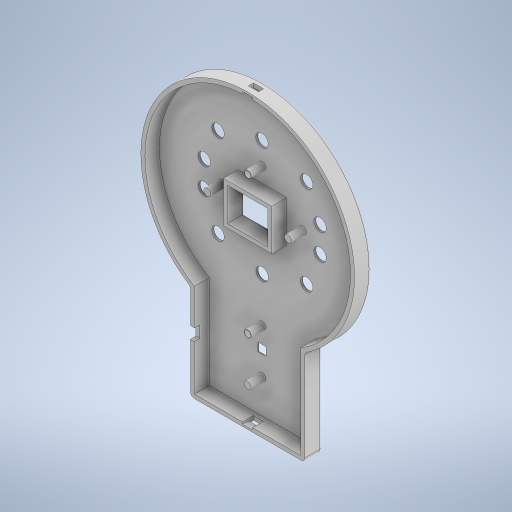
# Autodesk Inventor part: TopBox
Saved by Autodesk Inventor 2024 (Build 280153000, 153)
## iProperties
Created: 2023-11-16
Part Number: TopBox
Material: Générique
Document SubType Name: Modeling
Designer: digiacom
Density: 1 g/cm^3
Appearance: Par défaut
Author: digiacom
Autodesk Inventor part; units mm, degrees
ref_plane "YZ Plane" through (0, 0, 0) normal (1, 0, 0) x (0, 1, 0)
ref_plane "XZ Plane" through (0, 0, 0) normal (0, 1, 0) x (-1, 0, 0)
ref_plane "XY Plane" through (0, 0, 0) normal (0, 0, 1) x (1, 0, 0)
sketch "Esquisse1" plane through (0, 0, 0) normal (0, 0, 1) x (1, 0, 0)
  circle A0 centre (0, 0) radius 51
  line L0 (0, 0) -> (-26.4, 0)
  line L1 (-26.4, 0) -> (-26.4, -90)
  line L2 (-26.4, -90) -> (0, -90)
  line L3 (0, -90) -> (0, 0)
  line L4 (0, 0) -> (26.4, 0)
  line L5 (26.4, 0) -> (26.4, -90)
  line L6 (26.4, -90) -> (0, -90)
  line L7 (0, -90) -> (0, 0)
  point P0 (26.4, -43.6353)
  point P1 (-26.4, -43.6353)
  dimension "d5" = 102
  dimension "d6" = 26.4
  dimension "d7" = 90
  dimension "d8" = 26.4
  constraints: 16 end point, 4 parallel, 2 horizontal, 2 perpendicular, 1 centre point, 1 coincident, 1 point on line
  measures "d5" diameter of A0
  measures "d6" distance of L2.end L1.end
  measures "d7" distance of L1.end L0.end
  measures "d8" distance of L5.end L6.end
extrude "Extrusion2" add sketch "Esquisse1" along normal blind 1
sketch "Esquisse2" plane through (0, 0, 1) normal (0, 0, 1) x (1, 0, 0)
  circle A0 centre (0, -50.9) radius 1.75
  line L0 (-26.4, -90) -> (26.4, -90) projected
  line L1 (-26.4, -43.6353) -> (-26.4, -90) projected
  circle A1 centre (0, 17.68) radius 1.75
  point P0 (0, 0)
  dimension "d11" = 3.5
  dimension "d12" = 39.1
  dimension "d13" = 26.4
  dimension "d19" = 3.5
  dimension "d20" = 107.68
  dimension "d21" = 26.4
  constraints: 2 centre point
  measures "d11" diameter of A0
  measures "d12" distance from line of L0 A0.centre
  measures "d13" distance from line of L1 A0.centre
  measures "d19" diameter of A1
  measures "d20" distance from line of L0 A1.centre
  measures "d21" distance from line of L1 A1.centre
extrude "Extrusion5" add sketch "Esquisse2" along normal blind 7.195
sketch "Esquisse4" plane through (0, -50.9, 8.195) normal (0, 0, 1) x (1, 0, 0)
  circle A0 centre (0, 0) radius 1.5
  point P0 (0, 50.9)
  dimension "d24" = 3
  constraints: 1 centre point
  measures "d24" diameter of A0
sketch "Esquisse5" plane through (0, 17.68, 8.195) normal (0, 0, 1) x (1, 0, 0)
  circle A0 centre (0, 0) radius 1.75 projected
  circle A1 centre (0, 0) radius 1.5
  point P0 (0, -17.68)
  dimension "d25" = 3
  constraints: 1 centre point, 1 coincident
  measures "d25" diameter of A1
extrude "Extrusion6" cut sketch "Esquisse4" against normal blind 3
extrude "Extrusion7" cut sketch "Esquisse5" against normal blind 3 contours A1
sketch "Esquisse6" plane through (0, 0, 1) normal (0, 0, 1) x (1, 0, 0)
  circle A0 centre (0, -73) radius 1.75
  line L0 (-26.4, -90) -> (26.4, -90) projected
  circle A1 centre (20, 0) radius 1.75
  circle A2 centre (-20, 0) radius 1.75
  point P0 (0, 0)
  dimension "d30" = 3.5
  dimension "d31" = 17
  dimension "d32" = 3.5
  dimension "d33" = 3.5
  dimension "d34" = 20
  dimension "d37" = 20
  constraints: 3 centre point
  measures "d30" diameter of A0
  measures "d31" distance from line of L0 A0.centre
  measures "d32" diameter of A1
  measures "d33" diameter of A2
  measures "d34" distance of point (0, 0) A1.centre
  measures "d37" distance of point (0, 0) A2.centre
extrude "Extrusion8" add sketch "Esquisse6" along normal blind 7.195
sketch "Esquisse8" plane through (0, 0, 0) normal (0, 0, -1) x (-1, 0, 0)
  circle A0 centre (0, 0) radius 53
  circle A1 centre (0, 0) radius 51
  line L0 (-26.4, -90) -> (-26.4, -43.6353) projected
  line L1 (-26.4, -90) -> (26.4, -90)
  line L2 (26.4, -90) -> (26.4, -35.4414)
  line L3 (26.4, -35.4414) -> (-26.4, -35.4414)
  line L4 (-26.4, -35.4414) -> (-26.4, -90)
  line L5 (-28.4, -92) -> (28.4, -92)
  line L6 (28.4, -92) -> (28.4, -28.7229)
  line L7 (28.4, -28.7229) -> (-28.4, -28.7229)
  line L8 (-28.4, -28.7229) -> (-28.4, -92)
  point P0 (26.4, -43.6353)
  point P1 (28.4, -44.7486)
  point P2 (-28.4, -44.7486)
  dimension "d39" = 102
  dimension "d38" = 106
  dimension "d40" = 2
  dimension "d41" = 2
  dimension "d42" = 2
  constraints: 16 end point, 4 parallel, 2 coincident, 2 horizontal, 2 perpendicular, 1 centre point, 2 other
  measures "d38" diameter of A0
  measures "d40" distance between parallel lines of L8 L0
  measures "d41" distance between parallel lines of L5 L1
  measures "d42" distance between parallel lines of L2 L6
extrude "Extrusion9" add sketch "Esquisse8" against normal blind 8.195 contours A0 L6 A1 L8 | L8 A1 L0 A0 | A0 L0 L1 L2 L6 L5 L8 | A0 L2 A1 L6
fillet "Congé1" radius 1 4 edges at (0, 53, 0) (28.4, -68.3743, 0) (0, -92, 0) (-28.4, -68.3743, 0)
fillet "Congé2" radius 2 8 edges at (28.0904, -44.5781, 0.2766) (28.4, -44.7486, 4.5975) (28.1071, -91.7071, 0.2929) (28.4, -92, 4.5975) (-28.1071, -91.7071, 0.2929) (-28.4, -92, 4.5975) (-28.0904, -44.5781, 0.2766) (-28.4, -44.7486, 4.5975)
sketch "Esquisse9" plane through (0, 0, 1) normal (0, 0, 1) x (1, 0, 0)
  circle A0 centre (0, -28.8) radius 3.05
  line L0 (26.4, -90) -> (-26.4, -90) projected
  circle A1 centre (22.085, -22.12) radius 3.05
  arc A2 (26.4, -43.6353) -> (-26.4, -43.6353) centre (0, 0) ccw projected
  line L1 (-50.095, 49.99) -> (50.095, 49.99)
  line L2 (50.095, 49.99) -> (50.095, -89)
  line L3 (50.095, -89) -> (-50.095, -89)
  line L4 (-50.095, -89) -> (-50.095, 49.99)
  arc A3 (29.2945, -44.1682) -> (-29.2945, -44.1682) centre (0, 0) ccw projected
  circle A4 centre (28.705, -6) radius 3.05
  circle A5 centre (28.705, 6.75) radius 3.05
  circle A6 centre (22.085, 22) radius 3.05
  circle A7 centre (-0.1, 28.6) radius 3.05
  circle A8 centre (-21.915, 21.89) radius 3.05
  circle A9 centre (-28.705, 6.25) radius 3.05
  circle A10 centre (-28.705, -6.5) radius 3.05
  circle A11 centre (-21.915, -22.32) radius 3.05
  point P0 (50.095, -19.505)
  dimension "d47" = 6.1
  dimension "d48" = 0
  dimension "d49" = 61.2
  dimension "d52" = 6.1
  dimension "d55" = 50.095
  dimension "d56" = 50.095
  dimension "d57" = 28.01
  dimension "d58" = 138.99
  dimension "d59" = 1
  dimension "d60" = -49.99
  dimension "d61" = 66.88
  dimension "d62" = 6.1
  dimension "d63" = 21.39
  dimension "d64" = 83
  dimension "d65" = 6.1
  dimension "d66" = 95.75
  dimension "d67" = 6.1
  dimension "d68" = 111
  dimension "d69" = 6.1
  dimension "d70" = 117.6
  dimension "d71" = 50.195
  dimension "d72" = 6.1
  dimension "d73" = 28.18
  dimension "d74" = 28.1
  dimension "d75" = 6.1
  dimension "d76" = 21.39
  dimension "d77" = 95.25
  dimension "d78" = 6.1
  dimension "d79" = 83.5
  dimension "d80" = 6.1
  dimension "d81" = 66.68
  constraints: 10 centre point, 8 end point, 2 parallel, 1 horizontal, 1 midpoint, 1 perpendicular
  measures "d47" diameter of A0
  measures "d48" horizontal distance of point (0, 0) A0.centre
  measures "d49" distance from line of L0 A0.centre
  measures "d52" diameter of A1
  measures "d55" horizontal distance of point (50.095, -19.505) A3.centre
  measures "d56" distance from line of point (0, 0) L4
  measures "d57" distance from line of L2 A1.centre
  measures "d58" distance between parallel lines of L3 L1
  measures "d59" distance between parallel lines of L0 L3
  measures "d60" distance from line of A2.centre L1
  measures "d61" distance from line of L3 A1.centre
  measures "d62" diameter of A4
  measures "d63" distance from line of L2 A4.centre
  measures "d64" distance from line of L3 A4.centre
  measures "d65" diameter of A5
  measures "d66" distance from line of L3 A5.centre
  measures "d67" diameter of A6
  measures "d68" distance from line of L3 A6.centre
  measures "d69" diameter of A7
  measures "d70" distance from line of L3 A7.centre
  measures "d71" distance from line of A7.centre L2
  measures "d72" diameter of A8
  measures "d73" distance from line of L4 A8.centre
  measures "d74" distance from line of A8.centre L1
  measures "d75" diameter of A9
  measures "d76" distance from line of L4 A9.centre
  measures "d77" distance from line of A9.centre L3
  measures "d78" diameter of A10
  measures "d79" distance from line of L0 A10.centre
  measures "d80" diameter of A11
  measures "d81" distance from line of L3 A11.centre
extrude "Extrusion10" cut sketch "Esquisse9" against normal blind 2 contours A0 | A1 | A4 | A5 | A6 | A7 | A8 | A9 | A10 | A11
sketch "Esquisse10" plane through (-28.4, -90, 1) normal (-1, 0, 0) x (0, 0, 1)
  point P0 (-1, 90)
sketch "Esquisse11" plane through (-28.4, -90, 1) normal (-1, 0, 0) x (0, 0, 1)
  line L0 (7.195, 46.3647) -> (7.195, 0) projected
  line L1 (7.195, 22.55) -> (4.495, 22.55)
  line L2 (4.495, 22.55) -> (4.495, 28.45)
  line L3 (4.495, 28.45) -> (7.195, 28.45)
  line L4 (7.195, 28.45) -> (7.195, 22.55)
  line L5 (7.195, 0) -> (0, 0) projected
  point P0 (-1, 90)
  point P1 (5.845, 28.45)
  point P2 (7.195, 28.45)
  dimension "d82" = 28.45
  dimension "d83" = 5.9
  dimension "d84" = 2.7
  constraints: 8 end point, 2 parallel, 1 horizontal, 1 midpoint, 1 perpendicular, 1 point on line
  measures "d82" distance between parallel lines of L3 L5
  measures "d83" distance from line of point (5.845, 28.45) L1
  measures "d84" distance between parallel lines of L0 L2
extrude "Extrusion11" cut sketch "Esquisse11" against normal blind 2
sketch "Esquisse12" plane through (0, 0, 0) normal (0, 0, -1) x (-1, 0, 0)
  line L0 (-1.9, -59.1) -> (2.1, -59.1)
  line L1 (2.1, -59.1) -> (2.1, -63.1)
  line L2 (2.1, -63.1) -> (-1.9, -63.1)
  line L3 (-1.9, -63.1) -> (-1.9, -59.1)
  line L4 (-28.4, -45.8349) -> (-28.4, -90) projected
  line L5 (-26.4, -92) -> (26.4, -92) projected
  point P0 (0, 0)
  point P1 (2.1, -61.1)
  point P2 (-1.9, -61.1)
  point P3 (0.1, -63.1)
  point P4 (0.1, -59.1)
  dimension "d87" = 4
  dimension "d88" = 26.5
  dimension "d89" = 4
  dimension "d90" = 28.9
  constraints: 8 end point, 4 midpoint, 2 parallel, 1 horizontal, 1 perpendicular
  measures "d87" distance from line of point (2.1, -61.1) L3
  measures "d88" distance from line of L4 point (-1.9, -61.1)
  measures "d89" distance of point (0.1, -63.1) point (0.1, -59.1)
  measures "d90" distance between parallel lines of L5 L2
extrude "Extrusion12" cut sketch "Esquisse12" against normal blind 1
fillet "Congé3" radius 1 4 edges at (1.9, -61.1, 0) (-0.1, -59.1, 0) (-0.1, -63.1, 0) (-2.1, -61.1, 0)
sketch "Esquisse13" plane through (-26.4, -92, 1) normal (0, -1, 0) x (1, 0, 0)
  line L0 (23.9, 4.317) -> (28.9, 4.317)
  line L1 (28.9, 4.317) -> (28.9, 1.817)
  line L2 (28.9, 1.817) -> (23.9, 1.817)
  line L3 (23.9, 1.817) -> (23.9, 4.317)
  line L4 (-2.8945, 7.195) -> (-2.8945, 0) projected
  line L5 (55.6945, 0) -> (55.6945, 7.195) projected
  line L6 (0, 7.195) -> (52.8, 7.195) projected
  point P0 (26.4, -1)
  point P1 (-2.8945, 3.5975)
  point P2 (23.9, 3.067)
  point P3 (55.6945, 3.5975)
  point P4 (26.4, 1.817)
  point P5 (26.4, 4.317)
  dimension "d94" = 26.7945
  dimension "d95" = 5
  dimension "d96" = 26.7946
  dimension "d97" = 2.5
  dimension "d98" = 2.878
  constraints: 8 end point, 5 midpoint, 2 parallel, 1 horizontal, 1 perpendicular
  measures "d94" horizontal distance of point (-2.895, 3.598) point (23.9, 3.067)
  measures "d95" distance between parallel lines of L1 L3
  measures "d96" distance from line of point (55.695, 3.598) L1
  measures "d97" distance of point (26.4, 1.817) point (26.4, 4.317)
  measures "d98" distance between parallel lines of L6 L0
extrude "Extrusion13" cut sketch "Esquisse13" against normal blind 2
sketch "Esquisse14" plane through (0, 0, 8.195) normal (0, 0, 1) x (1, 0, 0)
  line L0 (-2.5, -90) -> (2.5, -90) projected
  line L1 (-2.5, -90) -> (2.5, -90)
  line L2 (2.5, -90) -> (2.5, -91)
  line L3 (2.5, -91) -> (-2.5, -91)
  line L4 (-2.5, -91) -> (-2.5, -90)
  point P0 (0, 0)
  dimension "d101" = 5
  dimension "d102" = 1
  constraints: 8 end point, 2 parallel, 1 horizontal, 1 perpendicular
  measures "d101" distance of L2.end L3.end
  measures "d102" distance of L1.end L2.end
extrude "Extrusion14" cut sketch "Esquisse14" against normal blind 3
sketch "Esquisse18" plane through (0, 0, 8.195) normal (0, 0, 1) x (1, 0, 0)
  arc A0 (26.4, -43.6353) -> (-26.4, -43.6353) centre (0, 0) ccw projected
  arc A1 (0, 51) -> (-2.4992, 50.9387) centre (0, 0) ccw
  arc A2 (2.4992, 50.9387) -> (0, 51) centre (0, 0) ccw
  line L0 (0, 51) -> (0, 52)
  arc A3 (27.4, -44.1955) -> (-27.4, -44.1955) centre (0, 0) ccw projected
  line L1 (0, 52) -> (2.5, 52) construction
  line L2 (-2.4992, 50.9387) -> (-2.5483, 51.9375)
  line L3 (2.4992, 50.9387) -> (2.5483, 51.9375)
  arc A4 (0, 52) -> (-2.5483, 51.9375) centre (0, 0) ccw
  arc A5 (2.5483, 51.9375) -> (0, 52) centre (0, 0) ccw
  point P0 (2.4992, 50.9387)
  dimension "d110" = 2.5
  dimension "d111" = 2.5
  dimension "d112" = 1
  dimension "d128" = 1
  dimension "d129" = 1
  constraints: 14 point on circle, 8 end point, 4 centre point, 2 concentric, 1 horizontal, 1 vertical
  measures "d110" distance of L0.start L2.start
  measures "d111" distance of L0.start L3.start
  measures "d112" distance of L0.start L0.end
  measures "d128" distance of L2.start L2.end
  measures "d129" distance of L3.start L3.end
ref_plane "Plan de construction7" through (0, 53, 0) normal (0, -1, 0) x (1, 0, 0)
sketch "Esquisse19" plane through (0, 53, 0) normal (0, -1, 0) x (1, 0, 0)
  line L0 (0, 5.317) -> (2.5, 5.317)
  line L1 (2.5, 5.317) -> (2.5, 2.817)
  line L2 (2.5, 2.817) -> (0, 2.817)
  line L3 (0, 2.817) -> (0, 5.317)
  line L4 (0, 5.317) -> (-2.5, 5.317)
  line L5 (-2.5, 5.317) -> (-2.5, 2.817)
  line L6 (-2.5, 2.817) -> (0, 2.817)
  line L7 (0, 2.817) -> (0, 5.317)
  line L8 (53, 8.195) -> (-53, 8.195) projected
  point P0 (0, 0)
  point P1 (29.2945, 8.195)
  point P2 (-29.2945, 8.195)
  dimension "d121" = 2.5
  dimension "d122" = 2.5
  dimension "d123" = 2.5
  dimension "d124" = 2.5
  dimension "d125" = 2.878
  constraints: 16 end point, 4 parallel, 2 horizontal, 2 perpendicular
  measures "d121" distance of L1.end L2.end
  measures "d122" distance of L0.end L1.end
  measures "d123" distance of L6.end L5.end
  measures "d124" distance of L5.end L4.end
  measures "d125" distance between parallel lines of L4 L8
extrude "Extrusion16" cut sketch "Esquisse19" along normal blind 7.122
extrude "Extrusion17" cut sketch "Esquisse18" against normal blind 2.878
sketch "Esquisse20" plane through (0, 0, 0) normal (0, 0, -1) x (-1, 0, 0)
  line L0 (-10, -8.5) -> (10, -8.5)
  line L1 (10, -8.5) -> (10, 8)
  line L2 (10, 8) -> (-10, 8)
  line L3 (-10, 8) -> (-10, -8.5)
  line L4 (-26.4, -92) -> (26.4, -92) projected
  line L5 (28.4, -90) -> (28.4, -45.8349) projected
  point P0 (0, 0)
  point P1 (0, -8.5)
  dimension "d132" = 83.5
  dimension "d133" = 20
  dimension "d134" = 16.5
  dimension "d135" = 18.4
  constraints: 8 end point, 2 parallel, 1 horizontal, 1 midpoint, 1 perpendicular
  measures "d132" distance between parallel lines of L4 L0
  measures "d133" distance between parallel lines of L1 L3
  measures "d134" distance from line of point (0, -8.5) L2
  measures "d135" distance between parallel lines of L5 L1
extrude "Extrusion18" cut sketch "Esquisse20" against normal blind 1
fillet "Congé4" radius 1 4 edges at (10, -0.25, 0) (0, 8, 0) (-10, -0.25, 0) (0, -8.5, 0)
sketch "Esquisse21" plane through (0, 0, 1) normal (0, 0, 1) x (1, 0, 0)
  line L0 (-12, -10.5) -> (12, -10.5)
  line L1 (12, -10.5) -> (12, 10)
  line L2 (12, 10) -> (-12, 10)
  line L3 (-12, 10) -> (-12, -10.5)
  line L4 (-10, -8.5) -> (-10, 8) projected
  line L5 (10, 8) -> (10, -8.5) projected
  line L6 (-10, 8) -> (10, 8) projected
  line L7 (10, -8.5) -> (-10, -8.5) projected
  point P0 (0, 0)
  dimension "d139" = 2
  dimension "d140" = 2
  dimension "d141" = 2
  dimension "d142" = 2
  constraints: 8 end point, 2 parallel, 1 horizontal, 1 perpendicular
  measures "d139" distance between parallel lines of L4 L3
  measures "d140" distance between parallel lines of L1 L5
  measures "d141" distance between parallel lines of L6 L2
  measures "d142" distance between parallel lines of L0 L7
extrude "Extrusion19" add sketch "Esquisse21" along normal blind 7.195
equation "\"d21\" = d13"
